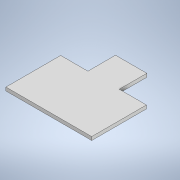
# Autodesk Inventor part: podstawa
Saved by Autodesk Inventor 2022 (Build 260153000, 153)
## iProperties
Created: 2022-12-08
Part Number: podstawa
Material: Generic
Document SubType Name: Modeling
Designer: Kamil
Density: 1 g/cm^3
Appearance: Default
Author: Kamil
Autodesk Inventor part; units mm, degrees
ref_plane "YZ Plane" through (0, 0, 0) normal (1, 0, 0) x (0, 1, 0)
ref_plane "XZ Plane" through (0, 0, 0) normal (0, 1, 0) x (-1, 0, 0)
ref_plane "XY Plane" through (0, 0, 0) normal (0, 0, 1) x (1, 0, 0)
sketch "Sketch1" plane through (0, 0, 0) normal (0, 1, 0) x (-1, 0, 0)
  line L0 (-49.6221, -50.9693) -> (50.3779, -50.9693)
  line L1 (50.3779, -50.9693) -> (50.3779, 49.0307)
  line L2 (50.3779, 49.0307) -> (-49.6221, 49.0307)
  line L3 (-49.6221, 49.0307) -> (-49.6221, -50.9693)
  line L4 (-17.8721, -0.5117) -> (18.6279, -0.5117)
  line L5 (18.6279, -0.5117) -> (18.6279, -50.9693)
  line L6 (18.6279, -50.9693) -> (-17.8721, -50.9693)
  line L7 (-17.8721, -50.9693) -> (-17.8721, -0.5117)
  line L8 (-49.6221, -18.7693) -> (50.3779, -18.7693)
  line L9 (50.3779, -18.7693) -> (50.3779, -50.9693)
  line L10 (50.3779, -50.9693) -> (-49.6221, -50.9693)
  line L11 (-49.6221, -50.9693) -> (-49.6221, -18.7693)
  line L12 (-49.6221, -18.7693) -> (50.3779, -18.7693)
  line L13 (50.3779, -18.7693) -> (50.3779, -14.7693)
  line L14 (50.3779, -14.7693) -> (-49.6221, -14.7693)
  line L15 (-49.6221, -14.7693) -> (-49.6221, -18.7693)
  line L16 (-49.6221, -34.8693) -> (50.3779, -34.8693)
  line L17 (-49.6221, -50.9693) -> (50.3779, -50.9693)
  line L18 (50.3779, -50.9693) -> (50.3779, -46.9693)
  line L19 (50.3779, -46.9693) -> (-49.6221, -46.9693)
  line L20 (-49.6221, -46.9693) -> (-49.6221, -50.9693)
  point P0 (0, 0)
  point P1 (0.3779, -50.9693)
  point P2 (0.3779, -50.9693)
  point P3 (0.3779, -50.9693)
  point P4 (-49.6221, -14.7693)
  point P5 (-17.8721, -14.7693)
  point P6 (-17.8721, -46.9693)
  point P7 (18.6279, -46.9693)
  point P8 (18.6279, -14.7693)
  dimension "d0" = 100
  dimension "d1" = 100
  dimension "d2" = 36.5
  dimension "d3" = 100
  dimension "d4" = 32.2
  dimension "d5" = 4
  dimension "d6" = 4
  constraints: 42 end point, 10 parallel, 5 horizontal, 5 midpoint, 5 perpendicular, 2 point on line
  measures "d0" distance of L2.end L1.end
  measures "d1" distance of L1.end L0.end
  measures "d2" distance of L5.end L6.end
  measures "d3" distance of L9.end L10.end
  measures "d4" distance of L8.end L9.end
  measures "d5" distance of L13.end L12.end
  measures "d6" distance of L18.end L17.end
extrude "Extrusion1" add sketch "Sketch1" along normal blind 4 contours L7 L16 L5 L19 | L7 L8 L5 L16 | L7 L14 L5 L8 | L3 L2 L1 L14 L5 L4 L7 | L7 L4 L5 L14
body "Solid1"
